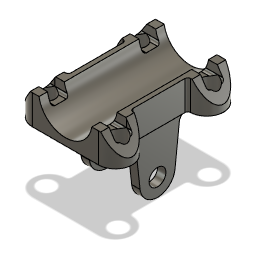
0.883.3681 - Demi-collier à chape pour tube 38 - IGTE 21465_204931 (Autodesk Fusion 360 design; units mm, degrees)
Autodesk Fusion 360 part; units mm, degrees
sketch "Sketch1" plane through (0, 0, 0) normal (0, 0, 1) x (1, 0, 0)
  line L0 (0, 0) -> (100, 0) construction
  line L1 (0, 0) -> (0, 50) construction
  line L2 (0, 0) -> (-100, 0) construction
  line L3 (0, -3) -> (-100, -3) construction
  line L4 (0, -3) -> (100, -3) construction
  line L5 (0, -24) -> (-100, -24) construction
  line L6 (15, -24) -> (100, -24) construction
  arc A0 (-22.9044, -3) -> (22.9044, -3) centre (0, 0) ccw construction
  arc A1 (-18.7617, -3) -> (18.7617, -3) centre (0, 0) ccw
  line L7 (25, 0) -> (25, 50) construction
  line L8 (-25, 0) -> (-25, 50) construction
  line L9 (-25, -3) -> (-25, -24) construction
  line L10 (-25, -24) -> (-35.5, -24)
  line L11 (-35.5, -24) -> (-35.5, -19)
  line L12 (-25, -3) -> (-18.7617, -3)
  line L13 (-35.5, -19) -> (-25, -3)
  line L14 (0, 0) -> (0, -100) construction
  line L15 (-15, 0) -> (-15, -100) construction
  line L16 (15, 0) -> (15, -100) construction
  line L17 (-21, 0) -> (-21, -100) construction
  line L18 (21, 0) -> (21, -100) construction
  line L19 (25, -24) -> (35.5, -24)
  line L20 (35.5, -24) -> (35.5, -19)
  line L21 (35.5, -19) -> (25, -3)
  line L22 (25, -3) -> (18.7617, -3)
  line L23 (0, -67.5) -> (-100, -67.5) construction
  line L24 (0, -67.5) -> (100, -67.5) construction
  line L25 (15, -67.5) -> (21, -67.5)
  line L26 (-21, -67.5) -> (-15, -67.5)
  line L27 (-15, -67.5) -> (-15, -29)
  line L28 (15, -29) -> (15, -67.5)
  line L29 (-10, -24) -> (10, -24)
  arc A2 (-10, -24) -> (-15, -29) centre (-10, -29) ccw
  arc A3 (15, -29) -> (10, -24) centre (10, -29) ccw
  line L30 (-21, -67.5) -> (-21, -24)
  line L31 (-25, -24) -> (-21, -24)
  line L32 (21, -24) -> (25, -24)
  line L33 (21, -24) -> (21, -67.5)
  dimension "d1" = 100
  dimension "d2" = 50
  dimension "d3" = 3
  dimension "d4" = 38
  dimension "d5" = 46.2
  dimension "d7" = 25
  dimension "d8" = 25
  dimension "d9" = 10.5
  dimension "d10" = 5
  dimension "d12" = 100
  dimension "d13" = 15
  dimension "d14" = 15
  dimension "d15" = 21
  dimension "d16" = 21
  dimension "d17" = 67.5
  dimension "d18" = 5
  dimension "d19" = 5
  constraint coincident L0.start L1.start
  constraint symmetric L0.start L1 L2.start
  constraint symmetric L0.end L1 L2.end
  constraint concentric A0 A1
  constraint coincident L3 A1.start
  constraint coincident L3 A0.start
  constraint coincident L4 A0.end
  constraint coincident L4 A1.end
  constraint coincident L5 L9.end
  constraint perpendicular L5 L9
  constraint coincident L3 L9.start
  constraint perpendicular L9 L12
  constraint symmetric A1.start L14 A1.end
  constraint symmetric L9.end L14 L19.start
  constraint symmetric L10.end L14 L19.end
  constraint symmetric L11.end L14 L20.end
  constraint symmetric L9.start L14 L21.end
  constraint coincident L24 L25.start
  constraint coincident L16 L25.start
  constraint coincident L24 L25.end
  constraint coincident L18 L25.end
  constraint perpendicular L18 L25
  constraint coincident L23 L26.start
  constraint coincident L17 L26.start
  constraint coincident L23 L26.end
  constraint coincident L15 L26.end
  constraint perpendicular L15 L26
  constraint coincident L16 L6.start
  constraint perpendicular L24 L28
  constraint perpendicular L16 L29
  constraint tangent L27 A2
  constraint tangent L29 A2
  constraint parallel L2 L5
  constraint parallel L0 L6
  constraint tangent L29 A3
  constraint tangent L28 A3
  constraint coincident L5 L30.end
  constraint coincident L17 L30.end
  constraint perpendicular L5 L30
  constraint coincident L6 L32.start
  constraint coincident L18 L32.start
  constraint perpendicular L18 L32
  constraint perpendicular L24 L33
  measures "d1" distance of L0.start L0.end
  measures "d2" distance of L0.start L1.end
  measures "d4" diameter of A1
  measures "d5" diameter of A0
  measures "d9" distance of L9.end L10.end
  measures "d12" distance of L0.start L14.end
  measures "d18" radius of A2
  measures "d19" radius of A3
extrude "Extrude1" add sketch "Sketch1" along normal mid plane 89 makes body 1
sketch "Sketch2" plane through (0, 0, 0) normal (1, 0, 0) x (0, 0, -1)
  line L0 (0, 0) -> (0, -55) construction
  line L1 (44.5, -3) -> (-44.5, -3) construction
  line L2 (-44.5, -3) -> (-44.5, -19) construction
  line L3 (-44.5, -19) -> (44.5, -19) construction
  line L4 (44.5, -19) -> (44.5, -3) construction
  line L5 (44.5, -19) -> (-44.5, -19) construction
  line L6 (-44.5, -19) -> (-44.5, -24) construction
  line L7 (-44.5, -24) -> (44.5, -24) construction
  line L8 (44.5, -24) -> (44.5, -19) construction
  line L9 (44.5, -24) -> (-44.5, -24) construction
  line L10 (-44.5, -24) -> (-44.5, -67.5) construction
  line L11 (-44.5, -67.5) -> (44.5, -67.5) construction
  line L12 (44.5, -67.5) -> (44.5, -24) construction
  circle A0 centre (0, -55) radius 6
  line L13 (-16, 0) -> (-16, -55) construction
  line L14 (16, 0) -> (16, -55) construction
  line L15 (15.5084, -28.4511) -> (12.4244, -56.3723)
  line L16 (-15.5084, -28.4511) -> (-12.4244, -56.3723)
  line L17 (20.4782, -24) -> (44.5, -24)
  line L18 (-44.5, -24) -> (-20.4782, -24)
  arc A1 (20.4782, -24) -> (15.5084, -28.4511) centre (20.4782, -29) ccw
  arc A2 (-15.5084, -28.4511) -> (-20.4782, -24) centre (-20.4782, -29) ccw
  arc A3 (-12.4244, -56.3723) -> (12.4244, -56.3723) centre (0, -55) ccw
  line L19 (0, -67.5) -> (44.5, -67.5)
  line L20 (0, -67.5) -> (-44.5, -67.5)
  line L21 (-44.5, -24) -> (-44.5, -67.5)
  line L22 (44.5, -24) -> (44.5, -67.5)
  line L23 (32.5, 0) -> (32.5, -55) construction
  line L24 (-32.5, 0) -> (-32.5, -55) construction
  line L25 (32.5, -3) -> (32.5, -11) construction
  line L26 (32.5, -11) -> (36.5, -11)
  line L27 (38.5, -9) -> (38.5, -3)
  line L28 (32.5, -11) -> (28.5, -11)
  line L29 (26.5, -9) -> (26.5, -3)
  line L30 (26.5, -3) -> (38.5, -3)
  arc A4 (36.5, -11) -> (38.5, -9) centre (36.5, -9) ccw
  arc A5 (26.5, -9) -> (28.5, -11) centre (28.5, -9) ccw
  line L31 (-38.5, -9) -> (-38.5, -3)
  arc A6 (-38.5, -9) -> (-36.5, -11) centre (-36.5, -9) ccw
  line L32 (-32.5, -11) -> (-36.5, -11)
  line L33 (-32.5, -11) -> (-28.5, -11)
  arc A7 (-28.5, -11) -> (-26.5, -9) centre (-28.5, -9) ccw
  line L34 (-26.5, -9) -> (-26.5, -3)
  line L35 (-26.5, -3) -> (-38.5, -3)
  point P0 (38.5, -11)
  dimension "d22" = 55
  dimension "d23" = 12
  dimension "d24" = 25
  dimension "d25" = 16
  dimension "d26" = 16
  dimension "d27" = 5
  dimension "d28" = 5
  dimension "d29" = 32.5
  dimension "d30" = 32.5
  dimension "d31" = 8
  dimension "d32" = 6
  dimension "d33" = 2
  constraint coincident L0.start origin
  constraint coincident L0.end A0.centre
  constraint concentric A0 A3
  constraint tangent L15 A3
  constraint tangent L16 A3
  constraint coincident L7.end L8.start
  constraint coincident L6.end L7.start
  constraint perpendicular L13 L18
  constraint tangent L17 A1
  constraint tangent L15 A1
  constraint tangent L16 A2
  constraint tangent L18 A2
  constraint midpoint A3 L19.start
  constraint coincident L11.end L12.start
  constraint tangent A3 L19
  constraint coincident L10.end L11.start
  constraint perpendicular L20 L21
  constraint coincident L23 L25.start
  constraint coincident L1 L25.start
  constraint coincident L1 L27.end
  constraint perpendicular L1 L27
  constraint symmetric L23 L25.end L26.start
  constraint symmetric L23 L27.end L29.end
  constraint perpendicular L27 L30
  constraint coincident P0 L26
  constraint coincident P0 L27
  constraint tangent L26 A4
  constraint tangent L27 A4
  constraint tangent L28 A5
  constraint tangent L29 A5
  constraint equal A4 A5
  constraint symmetric L0 L25.end L32.start
  constraint symmetric L0 L27.end L31.end
  constraint symmetric L0 L29.end L34.end
  constraint symmetric L0 L26.end A6.end
  constraint symmetric L0 L27.start L31.start
  constraint symmetric L0 A4 A6
  constraint symmetric L0 L28.end L33.end
  constraint symmetric L0 L29.start A7.end
  constraint symmetric L0 A5 A7
  measures "d22" distance of L0.start L0.end
  measures "d23" diameter of A0
  measures "d24" diameter of A3
  measures "d27" radius of A1
  measures "d28" radius of A2
  measures "d31" distance of L25.start L25.end
  measures "d32" distance of L25.end P0
  measures "d33" radius of A4
extrude "Extrude2" cut sketch "Sketch2" along normal through all and the other way through all bodies 1
sketch "Sketch3" plane through (0, 0, 0) normal (0, 1, 0) x (1, 0, 0)
  line L0 (-35.5, 44.5) -> (-35.5, -44.5) construction
  line L1 (-18.7617, 44.5) -> (18.7617, 44.5) construction
  line L2 (18.7617, -44.5) -> (-18.7617, -44.5) construction
  line L3 (35.5, 44.5) -> (35.5, -44.5) construction
  line L4 (35.5, -44.5) -> (25, -44.5) construction
  line L5 (25, -44.5) -> (18.7617, -44.5) construction
  line L6 (-18.7617, -44.5) -> (-25, -44.5) construction
  line L7 (-25, -44.5) -> (-35.5, -44.5) construction
  line L8 (-35.5, 44.5) -> (-25, 44.5) construction
  line L9 (-25, 44.5) -> (-18.7617, 44.5) construction
  line L10 (18.7617, 44.5) -> (25, 44.5) construction
  line L11 (25, 44.5) -> (35.5, 44.5) construction
  line L12 (35.5, 0) -> (-35.5, 0) construction
  line L13 (0, 44.5) -> (0, -44.5) construction
  line L14 (35.5, -44.5) -> (23.5, -44.5)
  line L15 (23.5, -44.5) -> (23.5, -32.5) construction
  line L16 (23.5, -32.5) -> (35.5, -32.5) construction
  line L17 (35.5, -32.5) -> (35.5, -44.5)
  line L18 (23.5, 32.5) -> (35.5, 32.5) construction
  line L19 (23.5, 44.5) -> (23.5, 32.5) construction
  line L20 (35.5, 32.5) -> (35.5, 44.5)
  line L21 (35.5, 44.5) -> (23.5, 44.5)
  line L22 (-23.5, 32.5) -> (-35.5, 32.5) construction
  line L23 (-23.5, 44.5) -> (-23.5, 32.5) construction
  line L24 (-23.5, -44.5) -> (-23.5, -32.5) construction
  line L25 (-23.5, -32.5) -> (-35.5, -32.5) construction
  line L26 (-35.5, 32.5) -> (-35.5, 44.5)
  line L27 (-35.5, 44.5) -> (-23.5, 44.5)
  line L28 (-35.5, -32.5) -> (-35.5, -44.5)
  line L29 (-35.5, -44.5) -> (-23.5, -44.5)
  line L30 (-23.5, -32.5) -> (-23.5, 32.5) construction
  line L31 (-22, -18.5089) -> (-22, 18.5089)
  line L32 (-23.5, 32.5) -> (23.5, 32.5) construction
  line L33 (-23.5, -32.5) -> (23.5, -32.5) construction
  line L34 (23.5, -32.5) -> (23.5, 32.5) construction
  arc A0 (-23.9286, -20.5077) -> (-23.5, -44.5) centre (-23.5, -32.5) ccw
  arc A1 (-23.5, 44.5) -> (-23.9286, 20.5077) centre (-23.5, 32.5) ccw
  arc A2 (23.9286, 20.5077) -> (23.5, 44.5) centre (23.5, 32.5) ccw
  arc A3 (23.5, -44.5) -> (23.9286, -20.5077) centre (23.5, -32.5) ccw
  arc A4 (-23.9286, -20.5077) -> (-22, -18.5089) centre (-24, -18.5089) ccw
  arc A5 (-22, 18.5089) -> (-23.9286, 20.5077) centre (-24, 18.5089) ccw
  line L35 (22, -18.5089) -> (22, 18.5089)
  arc A6 (23.9286, 20.5077) -> (22, 18.5089) centre (24, 18.5089) ccw
  arc A7 (22, -18.5089) -> (23.9286, -20.5077) centre (24, -18.5089) ccw
  line L36 (-35.5, -32.5) -> (-35.5, 32.5)
  line L37 (35.5, 32.5) -> (35.5, -32.5)
  line L38 (23.5, -32.5) -> (25.5, -32.4998)
  circle A8 centre (25.5, -32.4998) radius 6
  circle A9 centre (-25.5, -32.4998) radius 6
  circle A10 centre (-25.5, 32.4998) radius 6
  circle A11 centre (25.5, 32.4998) radius 6
  dimension "d36" = 12
  dimension "d37" = 12
  dimension "d38" = 24
  dimension "d40" = 2
  dimension "d41" = 2
  dimension "d42" = 2
  dimension "d43" = 2
  dimension "d46" = 2
  dimension "d47" = 12
  constraint midpoint L3 L12.start
  constraint midpoint L0 L12.end
  constraint midpoint L1 L13.start
  constraint midpoint L2 L13.end
  constraint horizontal L14
  constraint vertical L15
  constraint horizontal L16
  constraint vertical L17
  constraint coincident L3.end L4.start
  constraint coincident L15.end L16.start
  constraint symmetric L12 L14.end L19.start
  constraint symmetric L12 L15.end L18.start
  constraint symmetric L12 L16.end L18.end
  constraint symmetric L12 A2 A3
  constraint symmetric L12 L3.end L3.start
  constraint symmetric L13 L14.end L24.start
  constraint symmetric L13 L15.end L24.end
  constraint symmetric L13 L16.end L25.end
  constraint symmetric L13 A0 A3
  constraint symmetric L13 L18.start L22.start
  constraint symmetric L13 A1 A2
  constraint symmetric L13 L18.end L22.end
  constraint symmetric L13 L19.start L23.start
  constraint symmetric L13 L3.end L0.end
  constraint symmetric L13 L3.start L0.start
  constraint coincident L24.end L25.start
  constraint coincident L22.start L23.end
  constraint coincident L18.start L19.end
  constraint perpendicular L31 L33
  constraint symmetric L13 L24.end L15.end
  constraint symmetric L13 L22.start L18.start
  constraint parallel L30 L31
  constraint tangent L31 A4
  constraint tangent A0 A4
  constraint tangent L31 A5
  constraint tangent A1 A5
  constraint tangent A2 A6
  constraint tangent L35 A6
  constraint tangent A3 A7
  constraint tangent L35 A7
  constraint coincident L38.end A8.centre
  constraint symmetric L13 A8 A9
  constraint symmetric L12 A8 A11
  constraint symmetric L12 A9 A10
  measures "d36" distance of L3.end L14.end
  measures "d37" distance of L3.end L16.end
  measures "d38" diameter of A3
  measures "d40" radius of A4
  measures "d41" radius of A5
  measures "d42" radius of A6
  measures "d43" radius of A7
  measures "d46" distance of L15.end L38.end
  measures "d47" diameter of A8
extrude "Extrude3" cut sketch "Sketch3" against normal through all bodies 1
sketch "Sketch - Calage 1" plane through (15, 0, 0) normal (-1, 0, 0) x (0, 0, 1)
  line L0 (12.4244, -56.3723) -> (15.4477, -29)
  line L1 (15.4477, -29) -> (-15.4477, -29)
  line L2 (-15.4477, -29) -> (-12.4244, -56.3723)
  arc A0 (-12.4244, -56.3723) -> (12.4244, -56.3723) centre (0, -55) ccw
  circle A1 centre (0, -55) radius 6
  circle A2 centre (0, -55) radius 6
  line L3 (-15.4477, -29) -> (15.4477, -29)
  line L4 (12.4244, -56.3723) -> (15.4477, -29)
  arc A3 (-12.4244, -56.3723) -> (12.4244, -56.3723) centre (0, -55) ccw
  line L5 (-15.4477, -29) -> (-12.4244, -56.3723)
sketch "Sketch - Calage 2" plane through (-15, 0, 0) normal (1, 0, 0) x (0, 0, -1)
  circle A0 centre (0, -55) radius 6
  line L0 (-15.4477, -29) -> (-12.4244, -56.3723)
  arc A1 (-12.4244, -56.3723) -> (12.4244, -56.3723) centre (0, -55) ccw
  line L1 (12.4244, -56.3723) -> (15.4477, -29)
  line L2 (15.4477, -29) -> (-15.4477, -29)
  line L3 (12.4244, -56.3723) -> (15.4477, -29)
  line L4 (15.4477, -29) -> (-15.4477, -29)
  line L5 (-15.4477, -29) -> (-12.4244, -56.3723)
  arc A2 (-12.4244, -56.3723) -> (12.4244, -56.3723) centre (0, -55) ccw
  circle A3 centre (0, -55) radius 6
extrude "Extrude4" add sketch "Sketch - Calage 2" along normal blind 1 separate body makes body 2
extrude "Extrude5" add sketch "Sketch - Calage 1" along normal blind 1 draft 1 separate body makes body 3
hidden bodies 2 3
equation "d4 = ( 19 * 2 ) * 1 mm"
equation "d5 = ( 23.1 * 2 ) * 1 mm"
equation "d20 = 65 mm + 24 mm"
equation "d24 = ( 12.5 * 2 ) * 1 mm"
named bodies: "Calage 1", "Calage 2"
